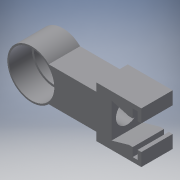
# Autodesk Inventor part: PistonV2
Saved by Autodesk Inventor 2016 (Build 200138000, 138)
## iProperties
Created: 2017-03-04
Part Number: PistonV2
Material: Generic
Document SubType Name: Modeling
Designer: Owner
Density: 1 g/cm^3
Appearance: Default
Author: Owner
Autodesk Inventor part; units mm, degrees
ref_plane "YZ Plane" through (0, 0, 0) normal (1, 0, 0) x (0, 1, 0)
ref_plane "XZ Plane" through (0, 0, 0) normal (0, 1, 0) x (-1, 0, 0)
ref_plane "XY Plane" through (0, 0, 0) normal (0, 0, 1) x (1, 0, 0)
sketch "Sketch1" plane through (0, 0, 0) normal (0, 1, 0) x (-1, 0, 0)
  line L0 (0, 0) -> (7, 0)
  line L1 (7, -23.495) -> (0, -23.495)
  line L2 (-11.75, -2) -> (-11.75, -21.5)
  line L3 (-11.75, -9.75) -> (-10, -9.75)
  line L4 (-10, -2) -> (-10, -21.5)
  line L5 (-11.75, -0.1283) -> (-10, -0.1283)
  line L6 (-10, -2) -> (-10, -6)
  line L7 (-11.75, -6) -> (-13.75, -6)
  line L8 (-13.75, -6) -> (-13.75, 0)
  line L9 (-10, -6) -> (-8, -6)
  line L10 (-8, -6) -> (-8, 0)
  line L11 (-8, 0) -> (-13.75, 0)
  line L12 (-10, -21.5) -> (-10, -17.5)
  line L13 (-10, -17.5) -> (-8, -17.5)
  line L14 (-8, -17.5) -> (-8, -23.5)
  line L15 (-10, -2) -> (-11.75, -2)
  line L16 (-11.75, -6) -> (-11.75, -2)
  line L17 (-10, -21.5) -> (-11.75, -21.5)
  line L18 (-11.75, -21.5) -> (-11.75, -17.5)
  line L19 (-11.75, -17.5) -> (-13.75, -17.5)
  line L20 (-13.75, -17.5) -> (-13.75, -23.5)
  line L21 (-13.75, -23.5) -> (-8, -23.5)
  line L22 (-0.01, -3.75) -> (7, -3.75)
  line L23 (-8, -6) -> (-0.01, -3.75)
  line L24 (-8, 0) -> (7, 0)
  line L25 (7, 0) -> (7, -3.75)
  line L26 (-8, -23.5) -> (7, -23.5)
  line L27 (7, -23.5) -> (7, -19.75)
  line L28 (7, -19.75) -> (-0.01, -19.75)
  line L29 (-8, -17.5) -> (-0.01, -19.75)
  line L30 (7, -23.5) -> (0, -23.5)
  line L31 (0, -23.5) -> (0, 0)
  line L32 (0, 0) -> (7, 0)
  line L33 (7, 0) -> (7, -23.5)
  line L34 (-10, -21.5) -> (-9.75, -21.5)
  line L35 (-9.75, -21.5) -> (-9.75, -17.5)
  line L36 (-9.75, -17.5) -> (-10, -17.5)
  line L37 (-10, -17.5) -> (-10, -21.5)
  line L38 (-11.75, -17.5) -> (-12, -17.5)
  line L39 (-12, -17.5) -> (-12, -21.5)
  line L40 (-12, -21.5) -> (-11.75, -21.5)
  line L41 (-11.75, -21.5) -> (-11.75, -17.5)
  line L42 (-10, -6) -> (-9.75, -6)
  line L43 (-9.75, -6) -> (-9.75, -2)
  line L44 (-9.75, -2) -> (-10, -2)
  line L45 (-10, -2) -> (-10, -6)
  line L46 (-11.75, -6) -> (-12, -6)
  line L47 (-12, -6) -> (-12, -2)
  line L48 (-12, -2) -> (-11.75, -2)
  line L49 (-11.75, -2) -> (-11.75, -6)
  dimension "d0" = 23.495
  dimension "d1" = 7
  dimension "d2" = 4
  dimension "d3" = 2
  dimension "d4" = 6
  dimension "d5" = 2
  dimension "d6" = 4
  dimension "d7" = 2
  dimension "d8" = 6
  dimension "d9" = 2
  dimension "d10" = 15
  dimension "d11" = 15
  dimension "d12" = 0.25
  dimension "d13" = 0.25
  dimension "d14" = 0.25
  dimension "d15" = 0.25
  constraints: 92 end point, 14 perpendicular, 11 parallel, 11 point on line, 8 horizontal, 2 coincident
  measures "d0" distance of L0.start L1.end
  measures "d1" distance of L0.start L0.end
  measures "d2" distance of L6.start L9.start
  measures "d3" distance of L16.start L7.end
  measures "d4" distance of L7.end L8.end
  measures "d5" distance of L9.start L9.end
  measures "d6" distance of L4.end L13.start
  measures "d7" distance of L13.start L29.start
  measures "d8" distance of L29.start L26.start
  measures "d9" distance of L19.start L19.end
  measures "d10" distance of L10.end L25.start
  measures "d11" distance of L26.start L26.end
  measures "d12" distance of L36.end L35.end
  measures "d13" distance of L40.end L39.end
  measures "d14" distance of L44.end L43.end
  measures "d15" distance of L47.end L48.end
extrude "Extrusion1" add sketch "Sketch1" along normal blind 14.5 contours L31 L22 L23 L10 L24 | L0 L25 L22 L31 | L10 L9 L43 L44 L15 L48 L47 L7 L8 L11 | L22 L33 L28 L31 | L31 L26 L14 L29 L28 | L28 L27 L1 L31 | L1 L27 L26 L31 | L14 L21 L20 L19 L39 L40 L17 L34 L35 L13
sketch "Sketch2" plane through (-7, 0, -23.5) normal (-1, 0, 0) x (0, 0, 1)
  line L0 (23.5, 0) -> (19.75, 0)
  line L1 (19.75, 0) -> (3.75, 0) projected
  line L2 (19.75, 0) -> (19.75, 14.5) projected
  line L3 (19.75, 0) -> (19.75, 14.5)
  line L4 (6, 0) -> (0, 0) projected
  line L5 (0, 0) -> (3.75, 0)
  line L6 (3.75, 0) -> (3.75, 14.5) projected
  line L7 (3.75, 0) -> (3.75, 14.5)
  line L8 (3.75, 0) -> (19.75, 0)
  line L9 (19.75, 0) -> (19.75, 14.5)
  line L10 (19.75, 14.5) -> (3.75, 14.5)
  line L11 (3.75, 14.5) -> (3.75, 0)
  dimension "d18" = 3.75
  dimension "d19" = 3.75
  constraints: 17 end point, 3 collinear, 2 parallel, 1 horizontal, 1 perpendicular
  measures "d18" distance of L0.start L0.end
  measures "d19" distance of L4.end L1.end
extrude "Extrusion2" add sketch "Sketch2" along normal blind 30
sketch "Sketch3" plane through (0, 0, 0) normal (0, -1, 0) x (1, 0, 0)
  line L0 (-37, -19.75) -> (-37, -3.75) projected
  circle A0 centre (-37, -11.75) radius 10.75
  point P0 (0, 0)
  dimension "d22" = 21.5
  constraints: 1 centre point, 1 midpoint
  measures "d22" diameter of A0
extrude "Extrusion3" add sketch "Sketch3" against normal blind 14.5
sketch "Sketch4" plane through (0, 0, 0) normal (0, -1, 0) x (1, 0, 0)
  arc A0 (-29.8193, -3.75) -> (-29.8193, -19.75) centre (-37, -11.75) ccw projected
  circle A1 centre (-37, -11.75) radius 10
  point P0 (0, 0)
  dimension "d25" = 20
  constraints: 1 centre point, 1 coincident
  measures "d25" diameter of A1
extrude "Extrusion4" cut sketch "Sketch4" against normal blind 10.5
sketch "Sketch5" plane through (-37, 10.5, -11.75) normal (0, -1, 0) x (1, 0, 0)
  circle A0 centre (0, 0) radius 10 projected
  circle A1 centre (0, 0) radius 9.5
  point P0 (37, 11.75)
  dimension "d28" = 19
  constraints: 1 centre point, 1 coincident
  measures "d28" diameter of A1
extrude "Extrusion5" cut sketch "Sketch5" against normal blind 10.5 contours A1
sketch "Sketch6" plane through (0, 0, -3.75) normal (1, 0, 0) x (0, 0, -1)
  circle A0 centre (8, 7.25) radius 5.25
  point P0 (-3.75, 0)
  dimension "d31" = 10.5
  constraints: 1 centre point
  measures "d31" diameter of A0
extrude "Extrusion6" cut sketch "Sketch6" against normal blind 40
sketch "Sketch7" plane through (0, 14.5, 0) normal (0, 1, 0) x (1, 0, 0)
  arc A0 (-29.8193, 19.75) -> (-29.8193, 3.75) centre (-37, 11.75) ccw projected
  circle A1 centre (-37, 11.75) radius 10.75
  point P0 (0, 0)
  dimension "d50" = 21.5
  constraints: 1 centre point, 1 coincident
  measures "d50" diameter of A1
extrude "Extrusion7" cut sketch "Sketch7" against normal blind 1
sketch "Sketch9" plane through (0, 0, 0) normal (0, -1, 0) x (1, 0, 0)
  line L0 (-7, -19.75) -> (-29.8193, -19.75) projected
  line L1 (-7, -19.75) -> (-4, -19.75)
  line L2 (-4, -19.75) -> (-4, -16.75)
  line L3 (-7, -3.75) -> (-7, 0) projected
  line L4 (-7, -3.75) -> (-4, -3.75)
  line L5 (-4, -3.75) -> (-4, -6.75)
  line L6 (-4, -16.75) -> (-24, -16.75)
  line L7 (-24, -16.75) -> (-24, -6.75)
  line L8 (-24, -6.75) -> (-4, -6.75)
  line L9 (-4, -6.75) -> (-4, -16.75)
  point P0 (0, 0)
  point P1 (-29.0904, -19.75)
  dimension "d39" = 3
  dimension "d40" = 3
  dimension "d41" = 3
  dimension "d42" = 3
  dimension "d43" = 20
  constraints: 16 end point, 3 horizontal, 2 parallel, 2 perpendicular, 1 vertical
  measures "d39" distance of L0.start L1.end
  measures "d40" distance of L1.end L2.end
  measures "d41" distance of L3.start L4.end
  measures "d42" distance of L4.end L5.end
  measures "d43" distance of L7.end L8.end
extrude "Extrusion9" cut sketch "Sketch9" against normal blind 3
sketch "Sketch10" plane through (0, 3, 0) normal (0, -1, 0) x (1, 0, 0)
  line L0 (-4, -8.6678) -> (-24, -8.6678) projected
  line L1 (-4, -6.75) -> (-4, -8.6678) projected
  line L2 (-24, -6.75) -> (-4, -6.75) projected
  line L3 (-24, -8.6678) -> (-24, -6.75) projected
  line L4 (-24, -14.8322) -> (-4, -14.8322) projected
  line L5 (-24, -16.75) -> (-24, -14.8322) projected
  line L6 (-4, -16.75) -> (-24, -16.75) projected
  line L7 (-4, -14.8322) -> (-4, -16.75) projected
  point P0 (0, 0)
extrude "Extrusion10" add sketch "Sketch10" along normal blind 3
sketch "Sketch11" plane through (13.75, 0, -17.5) normal (1, 0, 0) x (0, 0, -1)
  line L0 (-15.5, 11.975) -> (4, 11.975) projected
  line L1 (4, 0) -> (4, 14.5) projected
  line L2 (4, 11.975) -> (4, 14.5)
  line L3 (4, 14.5) -> (-15.625, 14.5)
  line L4 (-13.75, 14.5) -> (-17.5, 14.5) projected
  line L5 (-15.5, 0) -> (-15.5, 14.5) projected
  line L6 (-15.5, 11.975) -> (-15.5, 14.5)
  line L7 (4, 11.975) -> (-15.5, 11.975)
  line L8 (-15.5, 14.5) -> (4, 14.5)
  point P0 (-17.5, 0)
  constraints: 10 end point, 2 collinear, 1 horizontal, 1 midpoint, 1 vertical
extrude "Extrusion11" add sketch "Sketch11" against normal blind 5.75
body "Solid1"
